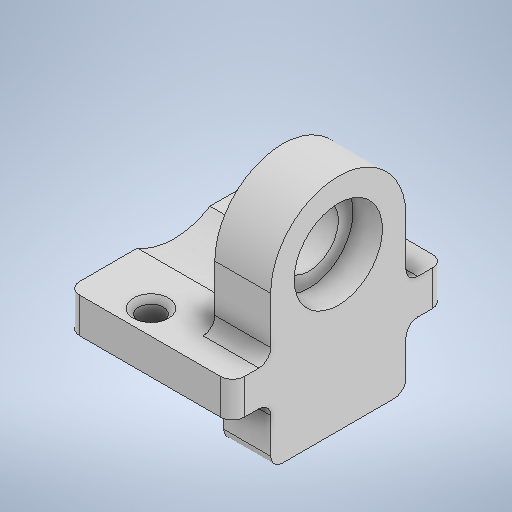
# Autodesk Inventor part: support_codeur
Saved by Autodesk Inventor 2025.2 (Build 292293000, 293)
## iProperties
Created: 2025-03-27
Part Number: support_codeur
Material: Générique
Document SubType Name: Modeling
Designer: enezl
Density: 1 g/cm^3
Appearance: Par défaut
Author: enezl
Autodesk Inventor part; units mm, degrees
ref_plane "YZ Plane" through (0, 0, 0) normal (1, 0, 0) x (0, 1, 0)
ref_plane "XZ Plane" through (0, 0, 0) normal (0, 1, 0) x (-1, 0, 0)
ref_plane "XY Plane" through (0, 0, 0) normal (0, 0, 1) x (1, 0, 0)
sketch "Esquisse1" plane through (0, 0, 0) normal (1, 0, 0) x (0, 1, 0)
  arc A0 (13, -11.5) -> (13, 11.5) centre (13, 0) ccw
  line L0 (-13, 11.5) -> (13, 11.5)
  line L1 (13, 11.5) -> (13, -11.5) construction
  line L2 (13, -11.5) -> (-13, -11.5)
  line L3 (-13, -11.5) -> (-13, 11.5)
  line L4 (-13, 11.5) -> (13, -11.5) construction
  line L5 (13, 11.5) -> (-13, -11.5) construction
  line L6 (-3, 11.5) -> (-3, -11.5)
  circle A1 centre (13, 0) radius 11.5 construction
  point P0 (0, 0)
  point P1 (0, 0)
  dimension "d1" = 23
  dimension "d2" = 16
  dimension "d3" = 10
  constraints: 14 end point, 3 midpoint, 2 centre point, 2 coincident, 2 parallel, 2 perpendicular, 2 point on circle, 2 point on line, 1 concentric, 1 horizontal, 1 tangent
  measures "d1" diameter of A0
  measures "d2" distance from line of L6 point (13, 0)
  measures "d3" distance between parallel lines of L6 L3
extrude "Extrusion1" add sketch "Esquisse1" along normal blind 8
extrude "Extrusion2" add sketch "Esquisse1" against normal blind 1.5 contours L2 L6 L0 A0
sketch "Esquisse3" plane through (8, 0, 0) normal (1, 0, 0) x (0, 0, -1)
  arc A0 (11.5, 13) -> (-11.5, 13) centre (0, 13) ccw projected
  point P0 (0, 0)
  point P1 (0, 13)
  constraints: 1 coincident
hole "Perçage1" at (8, 13, 0) direction (-1, 0, 0) diameter 10 end through all counterbore diameter 15 counterbore depth 5
sketch "Esquisse4" plane through (-1.5, 0, 0) normal (-1, 0, 0) x (0, 0, 1)
  circle A0 centre (0, 13) radius 5 projected
  circle A1 centre (0, 13) radius 8.5 construction
  circle A2 centre (0, 13) radius 7.5 projected
  point P0 (0, 0)
  point P1 (-8.5, 13)
  point P2 (7.5, 13)
  dimension "d15" = 17
  constraints: 2 horizontal alignment, 1 coincident, 3 other
hole "Perçage2" at (-1.5, 13, -8.5) at (-1.5, 13, 7.5) direction (1, 0, 0) diameter 3.2 depth 4
sketch "Esquisse5" plane through (8, 0, 0) normal (1, 0, 0) x (0, 0, -1)
  line L0 (18, 3) -> (-18, 3)
  line L1 (-18, 3) -> (-18, -3)
  line L2 (-18, -3) -> (18, -3)
  line L3 (18, -3) -> (18, 3)
  line L4 (18, 3) -> (-18, -3) construction
  line L5 (-18, 3) -> (18, -3) construction
  line L6 (11.5, -13) -> (11.5, 13) construction
  line L7 (11.5, -3) -> (-11.5, -3) projected
  point P0 (0, 0)
  dimension "d23" = 6.5
  constraints: 12 end point, 2 midpoint, 2 parallel, 1 collinear, 1 horizontal, 1 perpendicular
  measures "d23" distance between parallel lines of L6 L3
extrude "Extrusion3" add sketch "Esquisse5" against normal blind 28
fillet "Congé1" radius 2 10 edges at (8, 0, 18) (-20, 0, 18) (3.25, 3, 11.5) (4, -3, 11.5) (4, -3, -11.5) (8, 0, -18) (3.25, 3, -11.5) (-20, 0, -18) (4, -13, -11.5) (4, -13, 11.5)
sketch "Esquisse6" plane through (8, 3, 16) normal (0, 1, 0) x (1, 0, 0)
  line L0 (-18, 29.8634) -> (-18, 2.1366) construction
  line L1 (-9.5, 11) -> (-9.5, 21) projected
  line L2 (-5, 11) -> (-5, 21) projected
  line L3 (-11.5, 29.5) -> (-11.5, 2.5) projected
  line L4 (-11.5, 16) -> (-28, 16) construction
  line L5 (-28, 32) -> (-28, 0) projected
  point P0 (-8, 16)
  point P1 (-18, 16)
  dimension "d27" = 10
  constraints: 4 end point, 3 midpoint, 2 coincident, 1 point on line, 1 vertical
  measures "d27" distance between parallel lines of L0 L5
hole "Perçage3" at (-10, 3, -13.8634) at (-10, 3, 13.8634) direction (0, -1, 0) diameter 4.2 end through all countersink diameter 6 countersink angle 90
sketch "Esquisse7" plane through (-1.5, 0, 0) normal (-1, 0, 0) x (0, 0, 1)
  circle A0 centre (0, 13) radius 11.75
  arc A1 (11.5, 13) -> (-11.5, 13) centre (0, 13) ccw construction
  point P0 (0, 0)
  dimension "d36" = 23.5
  constraints: 1 centre point, 1 concentric
  measures "d36" diameter of A0
extrude "Extrusion4" cut sketch "Esquisse7" along normal through all
